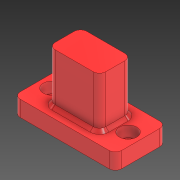
# Autodesk Inventor part: CH_01_0032_syringe_pump_needle_mount_2
Saved by Autodesk Inventor 2022 (Build 260153000, 153)
## iProperties
Created: 2022-04-21
Part Number: CH_01_0032_syringe_pump_needle_mount_2
Material: ABS Plastic
Document SubType Name: Modeling
Designer: Tomasz Krakowski
Density: 1.06 g/cm^3
Appearance: Light Red
Author: Tomasz Krakowski
Autodesk Inventor part; units mm, degrees
ref_plane "YZ Plane" through (0, 0, 0) normal (1, 0, 0) x (0, 1, 0)
ref_plane "XZ Plane" through (0, 0, 0) normal (0, 1, 0) x (-1, 0, 0)
ref_plane "XY Plane" through (0, 0, 0) normal (0, 0, 1) x (1, 0, 0)
sketch "Sketch1" plane through (0, 0, 0) normal (0, 1, 0) x (-1, 0, 0)
  line L0 (-14, 8) -> (14, 8)
  line L1 (16, 6) -> (16, -6)
  line L2 (14, -8) -> (-14, -8)
  line L3 (-16, -6) -> (-16, 6)
  line L4 (-16, 8) -> (16, -8) construction
  line L5 (16, 8) -> (-16, -8) construction
  arc A0 (16, 6) -> (14, 8) centre (14, 6) ccw
  arc A1 (14, -8) -> (16, -6) centre (14, -6) ccw
  arc A2 (-14, 8) -> (-16, 6) centre (-14, 6) ccw
  arc A3 (-16, -6) -> (-14, -8) centre (-14, -6) ccw
  circle A4 centre (-2, 0) radius 3.25
  line L6 (-2, 0) -> (0, 0) construction
  line L7 (0.5617, 2) -> (1.5333, 1.875)
  arc A5 (1.5333, -1.875) -> (1.5333, 1.875) centre (-2, 0) ccw
  line L8 (0.5617, -2) -> (1.5333, -1.875)
  line L9 (-2, 0) -> (-2, 3.25) construction
  line L10 (-4.5617, 2) -> (-5.5333, 1.875)
  arc A6 (-5.5333, 1.875) -> (-5.5333, -1.875) centre (-2, 0) ccw
  line L11 (-4.5617, -2) -> (-5.5333, -1.875)
  point P0 (-4, 0)
  point P1 (-4, 0)
  dimension "d0" = 32
  dimension "d1" = 16
  dimension "d2" = 2
  dimension "d3" = 6.5
  dimension "d48" = 14
  dimension "d49" = 4
  dimension "d50" = 1.875
  dimension "d51" = 2
  constraints: 24 end point, 14 point on circle, 8 point on line, 8 symmetric about line, 8 tangent, 7 centre point, 4 midpoint, 3 equal radius, 2 horizontal, 2 parallel, 1 coincident, 1 perpendicular, 1 vertical, 1 other
  measures "d0" distance between parallel lines of L3 L1
  measures "d1" distance between parallel lines of L0 L2
  measures "d2" radius of A0
  measures "d3" diameter of A4
  measures "d48" distance from line of L6.start L3
  measures "d49" radius of A5
  measures "d50" distance from line of L6 L7.end
  measures "d51" distance from line of L6 L7.start
extrude "Extrusion1" add sketch "Sketch1" along normal blind 1
sketch "Sketch2" plane through (0, 1, 0) normal (0, 1, 0) x (1, 0, 0)
  line L0 (6, -5) -> (-6, -5)
  line L1 (-8, -3) -> (-8, 3)
  line L2 (-6, 5) -> (6, 5)
  line L3 (8, 3) -> (8, -3)
  line L4 (8, -5) -> (-8, 5) construction
  line L5 (-8, -5) -> (8, 5) construction
  line L6 (-14, -8) -> (14, -8) construction
  line L7 (-16, 6) -> (-16, -6) construction
  arc A0 (-8, -3) -> (-6, -5) centre (-6, -3) ccw
  arc A1 (-6, 5) -> (-8, 3) centre (-6, 3) ccw
  arc A2 (8, 3) -> (6, 5) centre (6, 3) ccw
  arc A3 (6, -5) -> (8, -3) centre (6, -3) ccw
  circle A4 centre (2, 0) radius 2
  line L8 (2, 0) -> (0, 0) construction
  dimension "d10" = 8
  dimension "d11" = 3
  dimension "d12" = 2
  dimension "d13" = 2
  dimension "d53" = 2
  dimension "d54" = 4
  constraints: 14 end point, 8 point on circle, 8 point on line, 8 tangent, 5 centre point, 2 equal radius, 2 horizontal, 2 midpoint, 2 parallel, 1 perpendicular
  measures "d10" distance between parallel lines of L1 L7
  measures "d11" distance between parallel lines of L6 L0
  measures "d12" radius of A0
  measures "d13" radius of A1
  measures "d53" distance of L8.end L8.start
  measures "d54" diameter of A4
extrude "Extrusion2" add sketch "Sketch2" along normal blind 20
sketch "Sketch3" plane through (0, 1, 0) normal (0, 1, 0) x (1, 0, 0)
  arc A0 (8, 3) -> (6, 5) centre (6, 3) ccw projected
  line L0 (8, 3) -> (8, -3) projected
  arc A1 (6, -5) -> (8, -3) centre (6, -3) ccw projected
  line L1 (6, -5) -> (-6, -5) projected
  arc A2 (-8, -3) -> (-6, -5) centre (-6, -3) ccw projected
  line L2 (-8, -3) -> (-8, 3) projected
  arc A3 (-6, 5) -> (-8, 3) centre (-6, 3) ccw projected
  line L3 (-6, 5) -> (6, 5) projected
  line L4 (14, 8) -> (-14, 8) projected
  arc A4 (-14, 8) -> (-16, 6) centre (-14, 6) ccw projected
  line L5 (-16, 6) -> (-16, -6) projected
  arc A5 (-16, -6) -> (-14, -8) centre (-14, -6) ccw projected
  line L6 (-14, -8) -> (14, -8) projected
  arc A6 (14, -8) -> (16, -6) centre (14, -6) ccw projected
  line L7 (16, -6) -> (16, 6) projected
  arc A7 (16, 6) -> (14, 8) centre (14, 6) ccw projected
  point P0 (0, 0)
extrude "Extrusion3" add sketch "Sketch3" along normal blind 4
sketch "Sketch4" plane through (0, 5, 0) normal (0, 1, 0) x (1, 0, 0)
  line L0 (0, 0) -> (-12, 0) construction
  line L1 (-16, 6) -> (-16, -6) construction
  line L2 (12, 0) -> (0, 0) construction
  line L3 (16, -6) -> (16, 6) construction
  dimension "d19" = 4
  dimension "d20" = 4
  constraints: 4 end point, 1 collinear, 1 horizontal
  measures "d19" distance from line of L1 L0.end
  measures "d20" distance from line of L3 L2.start
hole "Hole1" at (-12, 5, 0) at (12, 5, 0) direction (0, -1, 0) diameter 3.5 end through all start extended yes counterbore diameter 5.5 counterbore depth 3.5
chamfer "Chamfer1" distance 1 angle 45 8 edges at (-8, 5, 0) (-7.4142, 5, 4.4142) (0, 5, 5) (7.4142, 5, 4.4142) (8, 5, 0) (7.4142, 5, -4.4142) (0, 5, -5) (-7.4142, 5, -4.4142)
sketch "Sketch5" plane through (6, 21, -5) normal (0, 0, -1) x (-1, 0, 0)
  line L0 (12, 0) -> (0, 0) construction
  line L1 (6, 0) -> (6, -7) construction
  line L2 (0, 0) -> (12, 0) projected
  point P0 (6, -21)
  dimension "d31" = 7
  constraints: 2 end point, 1 midpoint, 1 perpendicular
  measures "d31" distance from line of L0 L1.end
hole "Hole2" at (0, 14, -5) direction (0, 0, 1) diameter 6.2 depth 6 start extended yes
sketch "Sketch6" plane through (0, 21, 0) normal (0, 1, 0) x (1, 0, 0)
  circle A0 centre (2, 0) radius 2 projected
extrude "Extrusion4" add sketch "Sketch6" against normal blind 3.75
body "Solid1"
